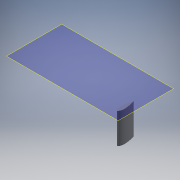
# Autodesk Inventor part: Tischbein
Saved by Autodesk Inventor 2017 (Build 210142000, 142)
## iProperties
Created: 2017-06-01
Part Number: Tischbein
Material: Generic
Document SubType Name: Modeling
Designer: Fake
Density: 1 g/cm^3
Appearance: Default
Author: Fake
Autodesk Inventor part; units mm, degrees
ref_plane "YZ Plane" through (0, 0, 0) normal (1, 0, 0) x (0, 1, 0)
ref_plane "XZ Plane" through (0, 0, 0) normal (0, 1, 0) x (-1, 0, 0)
ref_plane "XY Plane" through (0, 0, 0) normal (0, 0, 1) x (1, 0, 0)
ref_plane "Arbeitsebene1" through (-999.8717, -181.0364, 259.6495) normal (0, 0, -1) x (-1, 0, 0)
sketch "Skizze1" plane through (-999.8717, -181.0364, 259.6495) normal (0, 0, -1) x (-1, 0, 0)
  line L0 (1000, 8.7386) -> (-1000, 8.7386) projected
  line L1 (1000, 8.7386) -> (1000, 1000) projected
  line L2 (1000, 1000) -> (-1000, 1000) projected
  line L3 (-1000, 8.7386) -> (-1000, 1000) projected
  line L4 (0, 8.7386) -> (0, 1000) construction
  line L5 (-1919.7574, 928.6075) -> (-1998.0452, 872.3432) construction
  line L6 (-1998.0452, 872.3432) -> (-1919.7574, 598.6335) construction
  spline S0 degree 2 poles (-1919.7574, 928.6075) (-1998.0452, 872.3432) (-1919.7574, 598.6335) knots 1 1 1 2 2 2
  line L7 (-1919.7574, 598.6335) -> (-1841.4695, 872.3432) construction
  line L8 (-1841.4695, 872.3432) -> (-1919.7574, 928.6075) construction
  spline S1 degree 2 poles (-1919.7574, 598.6335) (-1841.4695, 872.3432) (-1919.7574, 928.6075) knots 1 1 1 2 2 2
  line L9 (-1919.7574, 598.6335) -> (-1919.7574, 928.6075) construction
  constraints: 4 end point, 2 midpoint, 1 symmetric about line, 1 vertical, 6 other
extrude "Extrusion1" add sketch "Skizze1" along normal blind 600 contours S1 S0
fillet "Rundung2" radius 9 1 edges at (919.8856, 417.5971, -40.3505)
